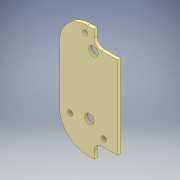
# Autodesk Inventor part: PCB Droit
Saved by Autodesk Inventor 2019 (Build 230136000, 136)
## iProperties
Created: 2018-06-08
Part Number: PCB Droit
Material: Nylon, disulfure de molybdène
Document SubType Name: Modeling
Designer: dimercur
Density: 1.13 g/cm^3
Appearance: Nylon 6
Mass: 2.24944 g
Surface Area: 27.2645 cm^2
Volume: 1.99065 cm^3
Author: dimercur
Autodesk Inventor part; units mm, degrees
ref_plane "YZ Plane" through (0, 0, 0) normal (1, 0, 0) x (0, 1, 0)
ref_plane "XZ Plane" through (0, 0, 0) normal (0, 1, 0) x (-1, 0, 0)
ref_plane "XY Plane" through (0, 0, 0) normal (0, 0, 1) x (1, 0, 0)
sketch "Esquisse1" plane through (0, 0, 0) normal (0, 1, 0) x (-1, 0, 0)
  line L0 (15.5, -30) -> (-15.5, -30)
  line L1 (-15.5, -30) -> (-15.5, 30)
  line L2 (-15.5, 30) -> (15.5, 30)
  line L3 (15.5, 30) -> (15.5, -30)
  point P0 (0, 0)
  dimension "d0" = 31
  dimension "d1" = 60
  dimension "d2" = 30
  dimension "d3" = 15.5
  constraints: 8 end point, 2 parallel, 1 horizontal, 1 perpendicular
  measures "d0" distance of L0.start L0.end
  measures "d1" distance of L2.end L0.start
  measures "d2" vertical distance of point (0, 0) L0.start
  measures "d3" horizontal distance of point (0, 0) L0.start
extrude "Extrusion1" add sketch "Esquisse1" along normal blind 1.6
fillet "Congé1" radius 15 2 edges at (-15.5, 0.8, -30) (-15.5, 0.8, 30)
sketch "Esquisse2" plane through (0, 1.6, 0) normal (0, 1, 0) x (1, 0, 0)
  circle A0 centre (7, 26) radius 4
  circle A1 centre (7, -26) radius 4
  line L0 (-0.5, -30) -> (15.5, -30) projected
  line L1 (3, 26) -> (3, 30)
  line L2 (15.5, 30) -> (-0.5, 30) projected
  line L3 (7, 30) -> (3, 30)
  line L4 (7, 30) -> (15.5, 30)
  line L5 (15.5, 30) -> (15.5, 22)
  line L6 (15.5, -30) -> (15.5, 30) projected
  line L7 (15.5, 22) -> (7, 22)
  line L8 (7, -22) -> (15.5, -22)
  line L9 (15.5, -22) -> (15.5, -30)
  line L10 (15.5, -30) -> (7, -30)
  line L11 (3, -26) -> (3, -30)
  line L12 (3, -30) -> (7, -30)
  point P0 (0, 0)
  dimension "d7" = 8
  dimension "d8" = 7
  dimension "d9" = 7
  dimension "d10" = 26
  dimension "d11" = 26
  constraints: 20 end point, 10 point on line, 8 point on circle, 2 centre point, 2 collinear, 2 tangent, 1 equal radius, 1 parallel, 1 perpendicular, 1 vertical
  measures "d7" diameter of A0
  measures "d8" horizontal distance of point (0, 0) A0.centre
  measures "d9" horizontal distance of point (0, 0) A1.centre
  measures "d10" vertical distance of point (0, 0) A0.centre
  measures "d11" vertical distance of point (0, 0) A1.centre
extrude "Extrusion3" cut sketch "Esquisse2" against normal through all
sketch "Esquisse3" plane through (0, 1.6, 0) normal (0, 1, 0) x (1, 0, 0)
  circle A0 centre (-9.75, 15) radius 1.3
  circle A1 centre (-1.75, -26) radius 1.3
  circle A2 centre (8.25, 18) radius 1.3
  line L0 (-15.5, 15) -> (-15.5, -15) projected
  circle A3 centre (2.689, -19.678) radius 2.5
  circle A4 centre (0.544, 12.678) radius 2.5
  point P0 (0, 0)
  dimension "d19" = 2.6
  dimension "d20" = 2.6
  dimension "d21" = 2.6
  dimension "d23" = 13.75
  dimension "d24" = 15
  dimension "d25" = 5.75
  dimension "d26" = 18
  dimension "d27" = 8.25
  dimension "d30" = 15.5
  dimension "d31" = 11
  dimension "d32" = 5
  dimension "d33" = 5
  dimension "d34" = 34.678
  dimension "d35" = 2.322
  dimension "d36" = 18.189
  dimension "d37" = 16.044
  constraints: 5 centre point
  measures "d19" diameter of A0
  measures "d20" diameter of A2
  measures "d21" diameter of A1
  measures "d23" distance from line of L0 A1.centre
  measures "d24" vertical distance of point (0, 0) A0.centre
  measures "d25" distance from line of L0 A0.centre
  measures "d26" vertical distance of point (0, 0) A2.centre
  measures "d27" horizontal distance of point (0, 0) A2.centre
  measures "d30" distance from line of L0 point (0, 0)
  measures "d31" vertical distance of A1.centre L0.end
  measures "d32" diameter of A3
  measures "d33" diameter of A4
  measures "d34" vertical distance of L0.start A3.centre
  measures "d35" vertical distance of L0.start A4.centre
  measures "d36" horizontal distance of A3.centre L0.start
  measures "d37" horizontal distance of L0.start A4.centre
extrude "Extrusion4" cut sketch "Esquisse3" against normal blind 18.189
equation "\"d2\" = 0.5 * d1"
equation "\"d3\" = 0.5 * d0"
equation "\"d9\" = d8"
equation "\"d11\" = d10"
equation "\"d20\" = d19"
equation "\"d21\" = d19"
equation "\"d33\" = d32"
equation "\"d28\" = d36"
